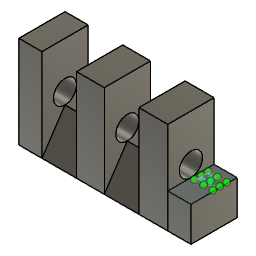
LogicUnit v2 (Autodesk Fusion 360 design; units mm, degrees)
Autodesk Fusion 360 part; units mm, degrees
note: some values were not read from the file. Set by a fixed rule: which sketch regions a step uses.
sketch "Sketch1" plane through (0, 0, 0) normal (0, 0, 1) x (1, 0, 0)
  line L0 (-66.04, 0) -> (-53.34, 0)
  line L1 (-53.34, 0) -> (-53.34, 25.4)
  line L2 (-53.34, 25.4) -> (-66.04, 25.4)
  line L3 (-66.04, 25.4) -> (-66.04, 0)
  line L4 (-34.29, 0) -> (-19.05, 0)
  line L5 (-19.05, 0) -> (-19.05, 25.4)
  line L6 (-19.05, 25.4) -> (-34.29, 25.4)
  line L7 (-34.29, 25.4) -> (-34.29, 0)
  line L8 (0, 0) -> (15.9232, 0)
  line L9 (15.9232, 0) -> (15.9232, 25.4)
  line L10 (15.9232, 25.4) -> (0, 25.4)
  line L11 (0, 25.4) -> (0, 0)
  dimension "d5" = 12.7
  dimension "d6" = 25.4
  dimension "d7" = 19.05
  dimension "d8" = 25.4
  dimension "d9" = 19.05
  dimension "d10" = 25.4
  constraint horizontal L0
  constraint vertical L1
  constraint horizontal L2
  constraint vertical L3
  constraint horizontal L4
  constraint vertical L5
  constraint horizontal L6
  constraint vertical L7
  constraint horizontal L8
  constraint vertical L9
  constraint horizontal L10
  constraint vertical L11
  measures "d5" distance of L0.start L0.end
  measures "d6" distance of L0.start L2.end
  measures "d7" distance of L1 L7
  measures "d8" distance of L4.start L6.end
  measures "d9" distance of L5 L11
  measures "d10" distance of L8.start L10.end
extrude "Extrude1" add sketch "Sketch1" along normal blind 50.8 makes body 1 at (0, 16.9333, 33.8667) makes body 2 at (-34.29, 16.9333, 33.8667) makes body 3 at (-66.04, 16.9333, 33.8667)
sketch "Sketch2" plane through (15.9232, 0, 0) normal (1, 0, 0) x (0, 1, 0)
  line L0 (0, 0) -> (25.4, 0)
  line L1 (25.4, 0) -> (25.4, 50.8)
  line L2 (25.4, 50.8) -> (0, 50.8)
  line L3 (0, 50.8) -> (0, 0)
  line L4 (12.7, 0) -> (12.7, 53.34)
  line L5 (25.4, 25.4) -> (-2.54, 25.4)
  circle A0 centre (12.7, 25.4) radius 6.35
  dimension "d15" = 12.7
  constraint midpoint L0 L4.start
  constraint perpendicular L2 L4
  constraint midpoint L1 L5.start
  constraint perpendicular L3 L5
  constraint coincident L5 A0.centre
  constraint coincident L4 A0.centre
  measures "d15" diameter of A0
extrude "Extrude2" cut sketch "Sketch2" against normal blind 96.52 contours L4 L5 A0 | L4 L5 A0 | L4 L5 A0 | L4 L5 A0 bodies 1 2 3
sketch "Sketch3" plane through (-53.34, 0, 0) normal (1, 0, 0) x (0, 1, 0)
  circle A0 centre (12.7, 25.4) radius 6.35
  line L0 (0, 0) -> (25.4, 0)
  line L1 (25.4, 0) -> (25.4, 50.8)
  line L2 (25.4, 50.8) -> (0, 50.8)
  line L3 (0, 50.8) -> (0, 0)
  line L4 (12.7, 25.4) -> (12.7, 0)
  line L5 (12.7, 19.05) -> (0, 0)
  line L6 (12.7, 19.05) -> (25.4, 0)
  line L7 (25.4, 0) -> (0, 0)
  constraint coincident A0.centre L4.start
  constraint midpoint L0 L4.end
  constraint coincident A0 L5.start
  constraint coincident L4 L5.start
  constraint coincident L0.start L3.end
  constraint coincident L0.end L1.start
extrude "Extrude3" add sketch "Sketch3" along normal blind 68.58 contours L0 L4 L6 L7 | L0 L4 L5 L7 bodies 1 2 3
sketch "Sketch4" plane through (15.9232, 0, 0) normal (1, 0, 0) x (0, 1, 0)
  circle A0 centre (12.7, 25.4) radius 6.35
  line L0 (0, 0) -> (25.4, 0)
  line L1 (25.4, 0) -> (25.4, 50.8)
  line L2 (25.4, 50.8) -> (0, 50.8)
  line L3 (0, 50.8) -> (0, 0)
  line L4 (12.7, 0) -> (12.7, 50.8)
  line L5 (12.7, 19.05) -> (0, 19.05)
  line L6 (12.7, 19.05) -> (25.4, 19.05)
  line L7 (0, 19.05) -> (25.4, 19.05)
  line L8 (25.4, 19.05) -> (25.4, 0)
  line L9 (25.4, 0) -> (0, 0)
  line L10 (0, 0) -> (0, 19.05)
  constraint midpoint L0 L4.start
  constraint midpoint L2 L4.end
  constraint coincident A0 L5.start
  constraint coincident L4 L5.start
  constraint coincident L3 L5.end
  constraint tangent A0 L5
  constraint coincident L1 L6.end
  constraint tangent A0 L6
  constraint horizontal L7
  constraint vertical L8
  constraint horizontal L9
  constraint vertical L10
  constraint coincident L0.end L1.start
extrude "Extrude4" add sketch "Sketch4" along normal blind 12.7 separate body contours L0 L1 L4 L6 L7 L8 L9 | L0 L3 L4 L5 L7 L9 L10 makes body 4
sketch "Sketch5" plane through (0, 0, 19.05) normal (0, 0, 1) x (-1, 0, 0)
  line L0 (-15.9232, -25.4) -> (-15.9232, 0)
  line L1 (-15.9232, 0) -> (-28.6232, 0)
  line L2 (-28.6232, 0) -> (-28.6232, -25.4)
  line L3 (-28.6232, -25.4) -> (-15.9232, -25.4)
  line L4 (-17.78, -12.7) -> (-27.94, -12.7) construction
  line L5 (-27.94, -12.7) -> (-27.94, -20.32) construction
  line L6 (-27.94, -20.32) -> (-17.78, -20.32) construction
  line L7 (-17.78, -20.32) -> (-17.78, -12.7) construction
  dimension "d23" = 2.54
equation "SorterLength = 1 in"
equation "SorterWidth = 0.5 in"
equation "WallWidth = SorterWidth * 1.2"
equation "WallLength = SorterLength * 1.2"
equation "d5 = SorterWidth"
equation "d6 = SorterLength"
equation "d7 = 1.5 * SorterWidth"
equation "d8 = SorterLength"
equation "d9 = 1.5 * SorterWidth"
equation "d10 = SorterLength"
equation "depth = 2 in"
equation "d12 = depth"
equation "AxleHoleDia = 0.5 in"
equation "d15 = AxleHoleDia"
